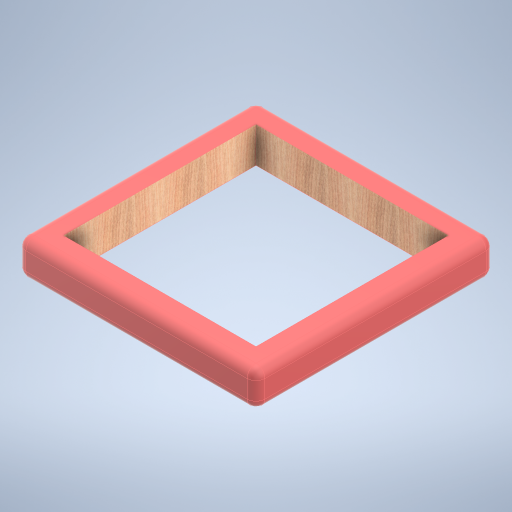
# Autodesk Inventor part: Bumpers
Saved by Autodesk Inventor 2024.2 (Build 282272000, 272)
## iProperties
RuleStatus: InUse
Created: 2024-01-14
Part Number: Bumpers
Material: Generic
Document SubType Name: Modeling
Designer: rohan
Density: 1 g/cm^3
Appearance: Smooth - Red
AfterAnyParamChange0: Bumper_Measurements
AfterAnyParamChange1: Bumper_Suppression
AfterAnyUserParamChange0: Bumper_Measurements
AfterAnyUserParamChange1: Bumper_Suppression
AfterFeatureSuppressionChange0: Bumper_Measurements
AfterFeatureSuppressionChange1: Bumper_Suppression
PartBodyChanged0: Bumper_Measurements
PartBodyChanged1: Bumper_Suppression
Author: rohan
Autodesk Inventor part; units mm, degrees
ref_plane "YZ Plane" through (0, 0, 0) normal (1, 0, 0) x (0, 1, 0)
ref_plane "XZ Plane" through (0, 0, 0) normal (0, 1, 0) x (-1, 0, 0)
ref_plane "XY Plane" through (0, 0, 0) normal (0, 0, 1) x (1, 0, 0)
sketch "Sketch1" plane through (0, 0, 0) normal (0, 1, 0) x (-1, 0, 0)
  line L0 (342.9, 342.9) -> (-342.9, 342.9)
  line L1 (-342.9, 342.9) -> (-342.9, -342.9)
  line L2 (-342.9, -342.9) -> (342.9, -342.9)
  line L3 (342.9, -342.9) -> (342.9, 342.9)
  line L4 (342.9, 342.9) -> (-342.9, -342.9) construction
  line L5 (-342.9, 342.9) -> (342.9, -342.9) construction
  line L6 (425.45, 425.45) -> (-425.45, 425.45)
  line L7 (-425.45, 425.45) -> (-425.45, -425.45)
  line L8 (-425.45, -425.45) -> (425.45, -425.45)
  line L9 (425.45, -425.45) -> (425.45, 425.45)
  line L10 (425.45, 425.45) -> (-425.45, -425.45) construction
  line L11 (-425.45, 425.45) -> (425.45, -425.45) construction
  point P0 (0, 0)
  dimension "d0" = 82.55
  dimension "d1" = 82.55
  dimension "d2" = 685.8
  dimension "d3" = 685.8
  constraints: 24 end point, 4 midpoint, 4 parallel, 2 horizontal, 2 perpendicular
  measures "d0" distance between parallel lines of L2 L8
  measures "d1" distance between parallel lines of L3 L9
  measures "d2" distance of L2.end L0.start
  measures "d3" distance of L0.start L0.end
extrude "Extrusion1" add sketch "Sketch1" along normal blind 127
fillet "Fillet1" radius 31.75 12 edges at (0, 127, 425.45) (0, 0, 425.45) (425.45, 63.5, 425.45) (425.45, 127, 0) (425.45, 0, 0) (425.45, 63.5, -425.45) (0, 127, -425.45) (-425.45, 127, 0) (-425.45, 63.5, 425.45) (0, 0, -425.45) (-425.45, 63.5, -425.45) (-425.45, 0, 0)
sketch "Bumper_Gaps" plane through (0, 127, 0) normal (0, 1, 0) x (1, 0, 0)
  line L0 (-203.2, -425.45) -> (203.2, -425.45)
  line L1 (203.2, -425.45) -> (203.2, -342.9)
  line L2 (203.2, -342.9) -> (-203.2, -342.9)
  line L3 (-203.2, -342.9) -> (-203.2, -425.45)
  line L4 (-203.2, -425.45) -> (203.2, -342.9) construction
  line L5 (203.2, -425.45) -> (-203.2, -342.9) construction
  line L6 (-425.45, -254) -> (-342.9, -254)
  line L7 (-342.9, -254) -> (-342.9, 254)
  line L8 (-342.9, 254) -> (-425.45, 254)
  line L9 (-425.45, 254) -> (-425.45, -254)
  line L10 (-425.45, -254) -> (-342.9, 254) construction
  line L11 (-342.9, -254) -> (-425.45, 254) construction
  line L12 (342.9, -254) -> (425.45, -254)
  line L13 (425.45, -254) -> (425.45, 254)
  line L14 (425.45, 254) -> (342.9, 254)
  line L15 (342.9, 254) -> (342.9, -254)
  line L16 (342.9, -254) -> (425.45, 254) construction
  line L17 (425.45, -254) -> (342.9, 254) construction
  line L18 (-342.9, -342.9) -> (-342.9, 342.9) projected
  line L19 (-425.45, 393.7) -> (-425.45, -393.7) projected
  line L20 (342.9, 342.9) -> (342.9, -342.9) projected
  line L21 (425.45, -393.7) -> (425.45, 393.7) projected
  line L22 (342.9, -342.9) -> (-342.9, -342.9) projected
  line L23 (-393.7, -425.45) -> (393.7, -425.45) projected
  line L24 (-196.85, 342.9) -> (196.85, 342.9)
  line L25 (196.85, 342.9) -> (196.85, 425.45)
  line L26 (196.85, 425.45) -> (-196.85, 425.45)
  line L27 (-196.85, 425.45) -> (-196.85, 342.9)
  line L28 (-196.85, 342.9) -> (196.85, 425.45) construction
  line L29 (196.85, 342.9) -> (-196.85, 425.45) construction
  line L30 (393.7, 425.45) -> (-393.7, 425.45) projected
  line L31 (-342.9, 342.9) -> (342.9, 342.9) projected
  point P0 (0, 0)
  point P1 (0, -384.175)
  point P2 (-384.175, 0)
  point P3 (384.175, 0)
  point P4 (0, 384.175)
  dimension "d15" = 406.4
  dimension "d16" = 393.7
  dimension "d17" = 508
  dimension "d18" = 508
  constraints: 48 end point, 8 collinear, 8 midpoint, 8 parallel, 4 horizontal, 4 perpendicular, 2 horizontal alignment, 2 vertical alignment
  measures "d15" distance between parallel lines of L1 L3
  measures "d16" distance between parallel lines of L25 L27
  measures "d17" distance between parallel lines of L14 L12
  measures "d18" distance between parallel lines of L8 L6
extrude "Front_Gap" [suppressed]
extrude "Back_Gap" [suppressed]
extrude "Left_Gap" [suppressed]
extrude "Right_Gap" [suppressed]
equation "\"d1\" = d0"
equation "\"d2\" = Length"
equation "\"d3\" = Width"
equation "\"d15\" = Front_Width"
equation "\"d16\" = Back_Width"
equation "\"d17\" = Left_Width"
equation "\"d18\" = Right_Width"
equation "\"Length\" = 685.8"
equation "\"Width\" = 685.8"
equation "\"Front_Width\" = 406.4"
equation "\"Back_Width\" = 393.7"
equation "\"Left_Width\" = 508"
equation "\"Right_Width\" = 508"
equation "\"Front_Edge\" = 152.4"
equation "\"Back_Edge\" = 152.4"
equation "\"Left_Edge\" = 152.4"
equation "\"Right_Edge\" = 152.4"
equation "\"FECalc\" = -0.5 * Front_Width + 0.5 * Width"
equation "\"BECalc\" = -0.5 * Back_Width + 0.5 * Width"
equation "\"LECalc\" = -0.5 * Left_Width + 0.5 * Length"
equation "\"RECalc\" = -0.5 * Right_Width + 0.5 * Length"
equation "\"FWCalc\" = Width - 2 * Front_Edge"
equation "\"BWCalc\" = Width - 2 * Back_Edge"
equation "\"LWCalc\" = Length - 2 * Left_Edge"
equation "\"RWCalc\" = Length - 2 * Right_Edge"
body "Solid1"
